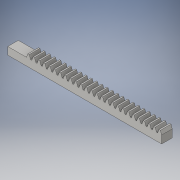
# Autodesk Inventor part: Lower Rack
Saved by Autodesk Inventor 2016 (Build 200138000, 138)
## iProperties
Created: 2016-04-02
Part Number: Lower Rack
Material: Generic
Document SubType Name: Modeling
Designer: amycroft3
Density: 1 g/cm^3
Appearance: Default
Author: amycroft3
Autodesk Inventor part; units mm, degrees
ref_plane "YZ Plane" through (0, 0, 0) normal (1, 0, 0) x (0, 1, 0)
ref_plane "XZ Plane" through (0, 0, 0) normal (0, 1, 0) x (-1, 0, 0)
ref_plane "XY Plane" through (0, 0, 0) normal (0, 0, 1) x (1, 0, 0)
sketch "Sketch1" plane through (0, 0, 0) normal (0, 0, 1) x (1, 0, 0)
  line L0 (27.3609, 9.329) -> (25.8428, 13.5)
  line L1 (25.8428, 13.5) -> (24.1571, 13.5)
  line L2 (24.1571, 13.5) -> (22.639, 9.329)
  arc A0 (22.1691, 9) -> (22.639, 9.329) centre (22.1691, 9.5) ccw
  line L3 (22.1691, 9) -> (0, 9)
  line L4 (0, 9) -> (0, 0)
  line L5 (103.5396, 9) -> (103.2289, 9)
  arc A1 (102.759, 9.329) -> (103.2289, 9) centre (103.2289, 9.5) ccw
  line L6 (102.759, 9.329) -> (101.2409, 13.5)
  line L7 (101.2409, 13.5) -> (99.5552, 13.5)
  line L8 (99.5552, 13.5) -> (98.0371, 9.329)
  arc A2 (97.5672, 9) -> (98.0371, 9.329) centre (97.5672, 9.5) ccw
  line L9 (97.5672, 9) -> (96.9457, 9)
  arc A3 (96.4759, 9.329) -> (96.9457, 9) centre (96.9457, 9.5) ccw
  line L10 (96.4759, 9.329) -> (94.9577, 13.5)
  line L11 (94.9577, 13.5) -> (93.272, 13.5)
  line L12 (93.272, 13.5) -> (91.7539, 9.329)
  arc A4 (91.2841, 9) -> (91.7539, 9.329) centre (91.2841, 9.5) ccw
  line L13 (91.2841, 9) -> (90.6625, 9)
  arc A5 (90.1927, 9.329) -> (90.6625, 9) centre (90.6625, 9.5) ccw
  line L14 (90.1927, 9.329) -> (88.6746, 13.5)
  line L15 (88.6746, 13.5) -> (86.9889, 13.5)
  line L16 (86.9889, 13.5) -> (85.4707, 9.329)
  arc A6 (85.0009, 9) -> (85.4707, 9.329) centre (85.0009, 9.5) ccw
  line L17 (85.0009, 9) -> (84.3794, 9)
  arc A7 (83.9095, 9.329) -> (84.3794, 9) centre (84.3794, 9.5) ccw
  line L18 (83.9095, 9.329) -> (82.3914, 13.5)
  line L19 (82.3914, 13.5) -> (80.7057, 13.5)
  line L20 (80.7057, 13.5) -> (79.1876, 9.329)
  arc A8 (78.7177, 9) -> (79.1876, 9.329) centre (78.7177, 9.5) ccw
  line L21 (78.7177, 9) -> (78.0962, 9)
  arc A9 (77.6263, 9.329) -> (78.0962, 9) centre (78.0962, 9.5) ccw
  line L22 (77.6263, 9.329) -> (76.1082, 13.5)
  line L23 (76.1082, 13.5) -> (74.4225, 13.5)
  line L24 (74.4225, 13.5) -> (72.9044, 9.329)
  arc A10 (72.4345, 9) -> (72.9044, 9.329) centre (72.4345, 9.5) ccw
  line L25 (72.4345, 9) -> (71.813, 9)
  arc A11 (71.3432, 9.329) -> (71.813, 9) centre (71.813, 9.5) ccw
  line L26 (71.3432, 9.329) -> (69.825, 13.5)
  line L27 (69.825, 13.5) -> (68.1393, 13.5)
  line L28 (68.1393, 13.5) -> (66.6212, 9.329)
  arc A12 (66.1514, 9) -> (66.6212, 9.329) centre (66.1514, 9.5) ccw
  line L29 (66.1514, 9) -> (65.5298, 9)
  arc A13 (65.06, 9.329) -> (65.5298, 9) centre (65.5298, 9.5) ccw
  line L30 (65.06, 9.329) -> (63.5419, 13.5)
  line L31 (63.5419, 13.5) -> (61.8562, 13.5)
  line L32 (61.8562, 13.5) -> (60.338, 9.329)
  arc A14 (59.8682, 9) -> (60.338, 9.329) centre (59.8682, 9.5) ccw
  line L33 (59.8682, 9) -> (59.2467, 9)
  arc A15 (58.7768, 9.329) -> (59.2467, 9) centre (59.2467, 9.5) ccw
  line L34 (58.7768, 9.329) -> (57.2587, 13.5)
  line L35 (57.2587, 13.5) -> (55.573, 13.5)
  line L36 (55.573, 13.5) -> (54.0549, 9.329)
  arc A16 (53.585, 9) -> (54.0549, 9.329) centre (53.585, 9.5) ccw
  line L37 (53.585, 9) -> (52.9635, 9)
  arc A17 (52.4936, 9.329) -> (52.9635, 9) centre (52.9635, 9.5) ccw
  line L38 (52.4936, 9.329) -> (50.9755, 13.5)
  line L39 (50.9755, 13.5) -> (49.2898, 13.5)
  line L40 (49.2898, 13.5) -> (47.7717, 9.329)
  arc A18 (47.3018, 9) -> (47.7717, 9.329) centre (47.3018, 9.5) ccw
  line L41 (47.3018, 9) -> (46.6803, 9)
  arc A19 (46.2105, 9.329) -> (46.6803, 9) centre (46.6803, 9.5) ccw
  line L42 (46.2105, 9.329) -> (44.6923, 13.5)
  line L43 (44.6923, 13.5) -> (43.0066, 13.5)
  line L44 (43.0066, 13.5) -> (41.4885, 9.329)
  arc A20 (41.0187, 9) -> (41.4885, 9.329) centre (41.0187, 9.5) ccw
  line L45 (41.0187, 9) -> (40.3971, 9)
  arc A21 (39.9273, 9.329) -> (40.3971, 9) centre (40.3971, 9.5) ccw
  line L46 (39.9273, 9.329) -> (38.4092, 13.5)
  line L47 (38.4092, 13.5) -> (36.7235, 13.5)
  line L48 (36.7235, 13.5) -> (35.2053, 9.329)
  arc A22 (34.7355, 9) -> (35.2053, 9.329) centre (34.7355, 9.5) ccw
  line L49 (34.7355, 9) -> (34.114, 9)
  arc A23 (33.6441, 9.329) -> (34.114, 9) centre (34.114, 9.5) ccw
  line L50 (33.6441, 9.329) -> (32.126, 13.5)
  line L51 (32.126, 13.5) -> (30.4403, 13.5)
  line L52 (30.4403, 13.5) -> (28.9222, 9.329)
  arc A24 (28.4523, 9) -> (28.9222, 9.329) centre (28.4523, 9.5) ccw
  line L53 (28.4523, 9) -> (27.8308, 9)
  arc A25 (27.3609, 9.329) -> (27.8308, 9) centre (27.8308, 9.5) ccw
  line L54 (0, 0) -> (103.5396, 0)
  line L55 (103.5396, 9) -> (103.5396, 0) construction
  line L56 (179.7184, 9.329) -> (181.2365, 13.5)
  line L57 (181.2365, 13.5) -> (182.9222, 13.5)
  line L58 (182.9222, 13.5) -> (184.4403, 9.329)
  arc A26 (103.8504, 9) -> (104.3203, 9.329) centre (103.8504, 9.5) ccw
  line L59 (103.5396, 9) -> (103.8504, 9)
  line L60 (104.3203, 9.329) -> (105.8384, 13.5)
  line L61 (105.8384, 13.5) -> (107.5241, 13.5)
  line L62 (107.5241, 13.5) -> (109.0422, 9.329)
  arc A27 (109.0422, 9.329) -> (109.5121, 9) centre (109.5121, 9.5) ccw
  line L63 (109.5121, 9) -> (110.1336, 9)
  arc A28 (110.1336, 9) -> (110.6034, 9.329) centre (110.1336, 9.5) ccw
  line L64 (110.6034, 9.329) -> (112.1216, 13.5)
  line L65 (112.1216, 13.5) -> (113.8073, 13.5)
  line L66 (113.8073, 13.5) -> (115.3254, 9.329)
  arc A29 (115.3254, 9.329) -> (115.7952, 9) centre (115.7952, 9.5) ccw
  arc A30 (116.4168, 9) -> (116.8866, 9.329) centre (116.4168, 9.5) ccw
  line L67 (115.7952, 9) -> (116.4168, 9)
  line L68 (129.453, 9.329) -> (130.9711, 13.5)
  line L69 (130.9711, 13.5) -> (132.6568, 13.5)
  line L70 (132.6568, 13.5) -> (134.1749, 9.329)
  arc A31 (134.1749, 9.329) -> (134.6448, 9) centre (134.6448, 9.5) ccw
  line L71 (134.6448, 9) -> (135.2663, 9)
  arc A32 (135.2663, 9) -> (135.7361, 9.329) centre (135.2663, 9.5) ccw
  line L72 (135.7361, 9.329) -> (137.2543, 13.5)
  line L73 (137.2543, 13.5) -> (138.94, 13.5)
  line L74 (138.94, 13.5) -> (140.4581, 9.329)
  arc A33 (140.4581, 9.329) -> (140.9279, 9) centre (140.9279, 9.5) ccw
  line L75 (140.9279, 9) -> (141.5495, 9)
  arc A34 (128.9831, 9) -> (129.453, 9.329) centre (128.9831, 9.5) ccw
  arc A35 (141.5495, 9) -> (142.0193, 9.329) centre (141.5495, 9.5) ccw
  line L76 (143.5374, 13.5) -> (145.2231, 13.5)
  line L77 (145.2231, 13.5) -> (146.7413, 9.329)
  arc A36 (146.7413, 9.329) -> (147.2111, 9) centre (147.2111, 9.5) ccw
  line L78 (147.2111, 9) -> (147.8326, 9)
  arc A37 (147.8326, 9) -> (148.3025, 9.329) centre (147.8326, 9.5) ccw
  line L79 (148.3025, 9.329) -> (149.8206, 13.5)
  line L80 (149.8206, 13.5) -> (151.5063, 13.5)
  line L81 (151.5063, 13.5) -> (153.0244, 9.329)
  arc A38 (153.0244, 9.329) -> (153.4943, 9) centre (153.4943, 9.5) ccw
  line L82 (153.4943, 9) -> (154.1158, 9)
  arc A39 (154.1158, 9) -> (154.5857, 9.329) centre (154.1158, 9.5) ccw
  line L83 (142.0193, 9.329) -> (143.5374, 13.5)
  line L84 (154.5857, 9.329) -> (156.1038, 13.5)
  line L85 (157.7895, 13.5) -> (159.3076, 9.329)
  arc A40 (159.3076, 9.329) -> (159.7775, 9) centre (159.7775, 9.5) ccw
  line L86 (159.7775, 9) -> (160.399, 9)
  arc A41 (160.399, 9) -> (160.8688, 9.329) centre (160.399, 9.5) ccw
  line L87 (160.8688, 9.329) -> (162.387, 13.5)
  line L88 (162.387, 13.5) -> (164.0727, 13.5)
  line L89 (164.0727, 13.5) -> (165.5908, 9.329)
  arc A42 (165.5908, 9.329) -> (166.0606, 9) centre (166.0606, 9.5) ccw
  line L90 (166.0606, 9) -> (166.6822, 9)
  arc A43 (166.6822, 9) -> (167.152, 9.329) centre (166.6822, 9.5) ccw
  line L91 (156.1038, 13.5) -> (157.7895, 13.5)
  line L92 (167.152, 9.329) -> (168.6701, 13.5)
  line L93 (168.6701, 13.5) -> (170.3558, 13.5)
  line L94 (170.3558, 13.5) -> (171.874, 9.329)
  arc A44 (171.874, 9.329) -> (172.3438, 9) centre (172.3438, 9.5) ccw
  line L95 (172.3438, 9) -> (172.9653, 9)
  arc A45 (172.9653, 9) -> (173.4352, 9.329) centre (172.9653, 9.5) ccw
  line L96 (173.4352, 9.329) -> (174.9533, 13.5)
  line L97 (174.9533, 13.5) -> (176.639, 13.5)
  line L98 (176.639, 13.5) -> (178.1571, 9.329)
  arc A46 (178.1571, 9.329) -> (178.627, 9) centre (178.627, 9.5) ccw
  line L99 (178.627, 9) -> (179.2485, 9)
  arc A47 (179.2485, 9) -> (179.7184, 9.329) centre (179.2485, 9.5) ccw
  line L100 (116.8866, 9.329) -> (118.4047, 13.5)
  line L101 (118.4047, 13.5) -> (120.0904, 13.5)
  line L102 (120.0904, 13.5) -> (121.6086, 9.329)
  arc A48 (121.6086, 9.329) -> (122.0784, 9) centre (122.0784, 9.5) ccw
  line L103 (122.0784, 9) -> (122.6999, 9)
  arc A49 (122.6999, 9) -> (123.1698, 9.329) centre (122.6999, 9.5) ccw
  line L104 (123.1698, 9.329) -> (124.6879, 13.5)
  line L105 (124.6879, 13.5) -> (126.3736, 13.5)
  line L106 (126.3736, 13.5) -> (127.8917, 9.329)
  arc A50 (127.8917, 9.329) -> (128.3616, 9) centre (128.3616, 9.5) ccw
  line L107 (128.3616, 9) -> (128.9831, 9)
  line L108 (184.4403, 0) -> (103.5396, 0)
  line L109 (184.4403, 9.329) -> (184.4403, 0)
  point P0 (87.8317, 5)
  point P1 (119.2476, 5)
  point P2 (207.0793, 0)
  dimension "d4" = 0.6215
  dimension "d5" = 0.3108
  constraints: 220 end point, 104 symmetric about line, 102 point on circle, 51 centre point, 2 perpendicular, 1 horizontal, 25 other
  measures "d4" distance of L9.start L9.end
  measures "d5" distance of L5.start L5.end
extrude "Extrusion1" add sketch "Sketch1" along normal blind 12.7
sketch "Sketch2" plane through (0, 0, 12.7) normal (0, 0, 1) x (1, 0, 0)
  line L0 (22.1691, 9) -> (0, 9) projected
  line L1 (175.6637, 9) -> (153.4945, 9) projected
  line L2 (0, 9) -> (175.6637, 9)
  point P0 (0, 0)
  constraints: 2 end point, 1 horizontal
equation "\"d5\" = 0.5 * d4"
body "Solid1"
